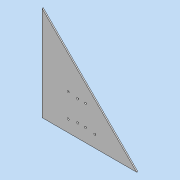
# Autodesk Inventor part: Display_CCM_Mount
Saved by Autodesk Inventor 2020 (Build 240168000, 168)
## iProperties
Created: 2021-07-12
Part Number: Display_CCM_Mount
Material: 一般
Document SubType Name: Sheet Metal
Designer: magnarecta
Density: 1 g/cm^3
Sheet Metal Rule: Default_mm
Appearance: 既定
Author: magnarecta
Autodesk Inventor part; units mm, degrees
ref_plane "YZ Plane" through (0, 0, 0) normal (1, 0, 0) x (0, 1, 0)
ref_plane "XZ Plane" through (0, 0, 0) normal (0, 1, 0) x (-1, 0, 0)
ref_plane "XY Plane" through (0, 0, 0) normal (0, 0, 1) x (1, 0, 0)
sketch "スケッチ1" plane through (0, 0, 0) normal (0, 0, 1) x (1, 0, 0)
  line L0 (0, 0) -> (239.9998, 0)
  line L1 (239.9998, 0) -> (239.9998, 239.9998)
  line L2 (239.9998, 239.9998) -> (0, 239.9998)
  line L3 (0, 239.9998) -> (0, 0)
  line L4 (0, 239.9998) -> (239.9998, 0)
  line L5 (-178.706, 178.706) -> (151.9787, -151.9787)
  dimension "d16" = 45
  dimension "d17" = 169.7055
  measures "d16" angle of L4 L0
  measures "d17" distance between parallel lines of L4 L5
extrude "プレート1" add sketch "スケッチ1" along normal blind 3 contours L3 L4 L0
sketch "スケッチ2" plane through (0, 0, 3) normal (0, 0, 1) x (1, 0, 0)
  line L0 (90, 33.5) -> (110, 33.5)
  line L1 (110, 33.5) -> (110, 86.5)
  line L2 (110, 86.5) -> (90, 86.5)
  line L3 (90, 86.5) -> (90, 33.5)
  line L4 (90, 33.5) -> (110, 86.5) construction
  line L5 (110, 33.5) -> (90, 86.5) construction
  line L6 (239.9998, 0) -> (0, 0) projected
  line L7 (0, 0) -> (0, 239.9998) projected
  line L8 (134, 30) -> (66, 30)
  line L9 (66, 30) -> (66, 90)
  line L10 (66, 90) -> (134, 90)
  line L11 (134, 90) -> (134, 30)
  line L12 (134, 30) -> (66, 90) construction
  line L13 (66, 30) -> (134, 90) construction
  point P0 (100, 60)
  dimension "d3" = 20
  dimension "d4" = 53
  dimension "d5" = 60
  dimension "d6" = 100
  dimension "d14" = 60
  dimension "d15" = 68
  constraints: 24 end point, 4 midpoint, 4 parallel, 2 horizontal, 2 perpendicular
  measures "d3" distance of L1.end L2.end
  measures "d4" distance of L0.end L1.end
  measures "d5" distance from line of point (100, 60) L6
  measures "d6" distance from line of point (100, 60) L7
  measures "d14" distance of L8.end L9.end
  measures "d15" distance of L8.start L8.end
hole "穴1" at (90, 33.5, 3) at (110, 33.5, 3) at (90, 86.5, 3) at (110, 86.5, 3) at (66, 30, 3) at (134, 30, 3) at (66, 90, 3) direction (0, 0, -1) diameter 5.2 depth 3 tip angle 118
equation "\"d12\" = Thickness"
equation "\"d2\" = Thickness"
equation "\"BendRadius\" = Thickness"
equation "\"BendReliefWidth\" = Thickness"
equation "\"BendReliefDepth\" = 0.5 * Thickness"
equation "\"CornerReliefSize\" = 4 * Thickness"
equation "\"MinimumRemnant\" = 2 * Thickness"
equation "\"TransitionRadius\" = BendRadius"
equation "\"JacobiRadiusSize\" = BendRadius"
equation "\"GapSize\" = Thickness"
equation "\"Thickness\" = 3"
